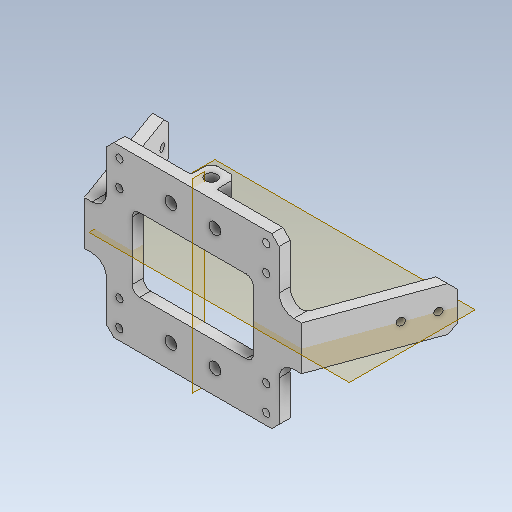
# Autodesk Inventor part: body_shell_2
Saved by Autodesk Inventor 2023 (Build 270158000, 158)
## iProperties
Created: 2021-03-01
Part Number: body_shell_2
Material: Generic
Document SubType Name: Modeling
Designer: Shuang Peng
Density: 1 g/cm^3
Appearance: Default
Author: Shuang Peng
Autodesk Inventor part; units mm, degrees
ref_plane "YZ Plane" through (0, 0, 0) normal (1, 0, 0) x (0, 1, 0)
ref_plane "XZ Plane" through (0, 0, 0) normal (0, 1, 0) x (-1, 0, 0)
ref_plane "XY Plane" through (0, 0, 0) normal (0, 0, 1) x (1, 0, 0)
sketch "Sketch1" plane through (0, 0, 0) normal (0, 0, 1) x (1, 0, 0)
  line L0 (-3.5, 39.5) -> (3.5, 39.5) projected
  line L1 (-3.5, 26.5) -> (-3.5, 39.5) projected
  line L2 (3.5, 26.5) -> (-3.5, 26.5) projected
  line L3 (3.5, 39.5) -> (3.5, 26.5) projected
  circle A0 centre (0, 36.5) radius 1.6 projected
  circle A1 centre (0, 29.5) radius 1.6 projected
  line L4 (-3.5, -6.5) -> (3.5, -6.5) projected
  line L5 (3.5, -6.5) -> (3.5, 6.5) projected
  line L6 (3.5, 6.5) -> (-3.5, 6.5) projected
  line L7 (-3.5, 6.5) -> (-3.5, -6.5) projected
  circle A2 centre (0, -3.5) radius 1.6 projected
  circle A3 centre (0, 3.5) radius 1.6 projected
  line L8 (-36.5, 39.5) -> (-43.5, 39.5) projected
  line L9 (-43.5, 39.5) -> (-43.5, 26.5) projected
  line L10 (-43.5, 26.5) -> (-36.5, 26.5) projected
  line L11 (-36.5, 26.5) -> (-36.5, 39.5) projected
  circle A4 centre (-40, 36.5) radius 1.6 projected
  circle A5 centre (-40, 29.5) radius 1.6 projected
  line L12 (-36.5, -6.5) -> (-43.5, -6.5) projected
  line L13 (-36.5, 6.5) -> (-36.5, -6.5) projected
  line L14 (-43.5, 6.5) -> (-36.5, 6.5) projected
  line L15 (-43.5, -6.5) -> (-43.5, 6.5) projected
  circle A6 centre (-40, -3.5) radius 1.6 projected
  circle A7 centre (-40, 3.5) radius 1.6 projected
  line L16 (3.5, 39.5) -> (-43.5, 39.5)
  line L17 (-43.5, 39.5) -> (-43.5, -6.5)
  line L18 (-43.5, -6.5) -> (3.5, -6.5)
  line L19 (3.5, -6.5) -> (3.5, 39.5)
  line L20 (-3.5, 26.5) -> (-36.5, 26.5)
  line L21 (-36.5, 26.5) -> (-36.5, 6.5)
  line L22 (-36.5, 6.5) -> (-3.5, 6.5)
  line L23 (-3.5, 6.5) -> (-3.5, 26.5)
  point P0 (0, 0)
  constraints: 16 end point, 4 parallel, 2 horizontal, 2 perpendicular
extrude "Extrusion1" add sketch "Sketch1" along normal blind 3 contours L0 L3 L2 L1 | L1 L20 L11 L16 | L2 L19 L6 L23 | L11 L10 L9 L8 | L21 L14 L17 L10 | L6 L5 L4 L7 | L7 L18 L13 L22 | L13 L12 L15 L14 | A0 | A1 | A2 | A3 | A4 | A5 | A6 | A7
sketch "Sketch2" plane through (0, 0, 3) normal (0, 0, 1) x (1, 0, 0)
  circle A0 centre (0, 36.5) radius 1 projected
  circle A1 centre (0, 29.5) radius 1 projected
  circle A2 centre (0, 3.5) radius 1 projected
  circle A3 centre (0, -3.5) radius 1 projected
  circle A4 centre (-40, -3.5) radius 1 projected
  circle A5 centre (-40, 3.5) radius 1 projected
  circle A6 centre (-40, 29.5) radius 1 projected
  circle A7 centre (-40, 36.5) radius 1 projected
  point P0 (0, 0)
hole "Hole1" at (0, 36.5, 3) at (0, 29.5, 3) at (0, 3.5, 3) at (0, -3.5, 3) at (-40, -3.5, 3) at (-40, 3.5, 3) at (-40, 29.5, 3) at (-40, 36.5, 3) direction (0, 0, -1) diameter 2 depth 20
ref_plane "Work Plane1" through (-20, -6.5, 0) normal (1, 0, 0) x (0, 0, -1)
sketch "Sketch3" plane through (0, 0, 0) normal (0, 0, -1) x (-1, 0, 0)
  circle A0 centre (40, 29.5) radius 1 projected
  circle A1 centre (40, -3.5) radius 1 projected
  circle A2 centre (0, 3.5) radius 1 projected
  circle A3 centre (0, 36.5) radius 1 projected
  circle A4 centre (0, 29.5) radius 1 projected
  circle A5 centre (0, -3.5) radius 1 projected
  circle A6 centre (40, 3.5) radius 1 projected
  circle A7 centre (40, 36.5) radius 1 projected
  line L0 (-3.5, 39.5) -> (43.5, 39.5) projected
  line L1 (-3.5, -6.5) -> (-3.5, 39.5) projected
  line L2 (43.5, -6.5) -> (-3.5, -6.5) projected
  line L3 (43.5, 39.5) -> (43.5, -6.5) projected
  line L4 (36.5, 26.5) -> (3.5, 26.5) projected
  line L5 (36.5, 6.5) -> (36.5, 26.5) projected
  line L6 (3.5, 6.5) -> (36.5, 6.5) projected
  line L7 (3.5, 26.5) -> (3.5, 6.5) projected
  line L8 (0.5, 22.5) -> (0.5, 10.5)
  line L9 (0.5, 10.5) -> (-7.5, 10.5)
  line L10 (-7.5, 10.5) -> (-7.5, 22.5)
  line L11 (-7.5, 22.5) -> (0.5, 22.5)
  line L12 (-3.5, -6.5) -> (-3.5, 39.5) projected
  line L13 (0.5, 22.5) -> (-7.5, 10.5) construction
  line L14 (0.5, 10.5) -> (-7.5, 22.5) construction
  point P0 (0, 0)
  point P1 (-3.5, 16.5)
  point P2 (-3.5, 10.5)
  point P3 (-3.5, 22.5)
  dimension "d9" = 12
  dimension "d10" = 8
  constraints: 12 end point, 3 midpoint, 2 parallel, 2 perpendicular
  measures "d9" distance of L8.start L8.end
  measures "d10" distance of L8.end L9.end
extrude "Extrusion2" add sketch "Sketch3" against normal up to surface (3 mm away) contours L1 L9 L10 L11
sketch "Sketch4" plane through (3.5, 10.5, 0) normal (0, -1, 0) x (1, 0, 0)
  line L0 (4, 3) -> (0, 3) projected
  line L1 (0, 0) -> (0, 3) projected
  line L2 (4, 0) -> (0, 0) projected
  line L3 (4, 0) -> (4, 3) projected
  line L4 (4, 0) -> (14.2606, -28.1908)
  line L5 (4, 3) -> (6.1006, 3)
  line L6 (6.1006, 3) -> (17.4531, -28.1908)
  line L7 (17.4531, -28.1908) -> (14.2606, -28.1908)
  point P0 (-3.5, 0)
  dimension "d13" = 30
  dimension "d14" = 110
  dimension "d15" = 3
  constraints: 8 end point, 2 parallel, 1 horizontal
  measures "d13" distance of L2.start L4.end
  measures "d14" angle of L2 L4
  measures "d15" distance between parallel lines of L4 L6
extrude "Extrusion3" add sketch "Sketch4" against normal up to surface (12 mm away) contours L5 L6 L7 L4 L3
ref_plane "Work Plane2" through (17.7606, 16.5, -28.1908) normal (0, 1, 0) x (1, 0, 0)
sketch "Sketch5" plane through (17.7606, 16.5, -28.1908) normal (0, 1, 0) x (1, 0, 0)
  line L0 (-58.7606, -28.1908) -> (-56.7606, -28.1908) projected
  line L1 (-58.7606, -28.1908) -> (-56.7606, -28.1908) projected
  line L2 (-18.7606, -28.1908) -> (-16.7606, -28.1908) projected
  line L3 (-18.7606, -28.1908) -> (-16.7606, -28.1908) projected
  line L4 (-18.7606, -28.1908) -> (-16.7606, -28.1908) projected
  line L5 (-18.7606, -28.1908) -> (-16.7606, -28.1908) projected
  line L6 (-58.7606, -28.1908) -> (-56.7606, -28.1908) projected
  line L7 (-58.7606, -28.1908) -> (-56.7606, -28.1908) projected
  line L8 (-14.2606, -28.1908) -> (-61.2606, -28.1908) projected
  line L9 (-61.2606, -28.1908) -> (-14.2606, -28.1908) projected
  line L10 (-54.2606, -28.1908) -> (-21.2606, -28.1908) projected
  line L11 (-21.2606, -28.1908) -> (-54.2606, -28.1908) projected
  line L12 (-10.2606, -28.1908) -> (0, 0) projected
  line L13 (-10.2606, -28.1908) -> (0, 0) projected
  line L14 (-10.2606, -28.1908) -> (-5.1303, -14.0954)
  line L15 (-21.2606, -28.1908) -> (-21.2606, -31.1908) projected
  line L16 (-5.1303, -14.0954) -> (-21.2606, -28.1908)
  line L17 (-14.2606, -28.1908) -> (-10.2606, -28.1908) projected
  line L18 (-10.2606, -28.1908) -> (-14.2606, -28.1908) projected
  point P0 (-17.7606, -28.1908)
  dimension "d19" = 15
  constraints: 4 end point, 1 midpoint
  measures "d19" distance of L14.start L14.end
extrude "Extrusion4" add sketch "Sketch5" along normal mid plane 2
mirror "Mirror1" about plane through (-20, -6.5, 0) normal (1, 0, 0) of "Extrusion2", "Extrusion3", "Extrusion4"
sketch "Sketch6" plane through (0, 0, 0) normal (0, 0, -1) x (-1, 0, 0)
  line L0 (36.5, 17.5) -> (47.5, 17.5) projected
  line L1 (47.5, 22.5) -> (47.5, 17.5) projected
  line L2 (43.5, 22.5) -> (47.5, 22.5) projected
  line L3 (43.5, 39.5) -> (43.5, 22.5) projected
  line L4 (-3.5, 39.5) -> (43.5, 39.5) projected
  line L5 (-3.5, 22.5) -> (-3.5, 39.5) projected
  line L6 (-3.5, 22.5) -> (-7.5, 22.5) projected
  line L7 (-7.5, 22.5) -> (-7.5, 17.5) projected
  line L8 (-7.5, 17.5) -> (3.5, 17.5) projected
  line L9 (3.5, 26.5) -> (3.5, 17.5) projected
  line L10 (36.5, 26.5) -> (3.5, 26.5) projected
  line L11 (36.5, 17.5) -> (36.5, 26.5) projected
  circle A0 centre (40, 29.5) radius 1 projected
  circle A1 centre (0, 36.5) radius 1 projected
  circle A2 centre (0, 29.5) radius 1 projected
  circle A3 centre (40, 36.5) radius 1 projected
  line L12 (47.5, 15.5) -> (36.5, 15.5) projected
  line L13 (36.5, 6.5) -> (36.5, 15.5) projected
  line L14 (3.5, 6.5) -> (36.5, 6.5) projected
  line L15 (3.5, 15.5) -> (3.5, 6.5) projected
  line L16 (3.5, 15.5) -> (-7.5, 15.5) projected
  line L17 (-7.5, 15.5) -> (-7.5, 10.5) projected
  line L18 (-7.5, 10.5) -> (-3.5, 10.5) projected
  line L19 (-3.5, -6.5) -> (-3.5, 10.5) projected
  line L20 (43.5, -6.5) -> (-3.5, -6.5) projected
  line L21 (43.5, 10.5) -> (43.5, -6.5) projected
  line L22 (47.5, 10.5) -> (43.5, 10.5) projected
  line L23 (47.5, 15.5) -> (47.5, 10.5) projected
  circle A4 centre (40, -3.5) radius 1 projected
  circle A5 centre (0, 3.5) radius 1 projected
  circle A6 centre (0, -3.5) radius 1 projected
  circle A7 centre (40, 3.5) radius 1 projected
  circle A8 centre (40, 36.5) radius 1 projected
  line L24 (40, 36.5) -> (40, 29.5)
  circle A9 centre (0, 36.5) radius 1 projected
  circle A10 centre (0, 29.5) radius 1 projected
  line L25 (0, 36.5) -> (0, 29.5)
  line L26 (40, 33) -> (0, 33)
  line L27 (20, 33) -> (14, 33)
  line L28 (20, 33) -> (26, 33)
  circle A11 centre (26, 33) radius 1.6
  circle A12 centre (14, 33) radius 1.6
  point P0 (0, 0)
  dimension "d23" = 6
  dimension "d24" = 6
  dimension "d25" = 3.2
  dimension "d26" = 3.2
  constraints: 10 end point, 3 midpoint, 2 centre point, 2 coincident, 2 vertical, 1 collinear, 1 point on line
  measures "d23" distance of L27.start L27.end
  measures "d24" distance of L27.start L28.end
  measures "d25" diameter of A11
  measures "d26" diameter of A12
extrude "Extrusion5" cut sketch "Sketch6" against normal blind 6 contours A11 L26 | L26 A11 | A12 L26 | L26 A12
mirror "Mirror2" about plane through (17.7606, 16.5, -28.1908) normal (0, 1, 0) of "Extrusion5"
sketch "Sketch7" plane through (-43.5, 39.5, 0) normal (0, 1, 0) x (1, 0, 0)
  line L0 (47, 0) -> (0, 0) projected
  line L1 (0, 0) -> (0, -3) projected
  line L2 (47, -3) -> (0, -3) projected
  line L3 (47, 0) -> (47, -3) projected
  line L4 (47, 0) -> (0, 0) projected
  line L5 (23.5, 0) -> (23.5, 2)
  line L6 (20, 5.5) -> (20, -1.5)
  line L7 (20, -1.5) -> (27, -1.5)
  line L8 (27, -1.5) -> (27, 5.5)
  line L9 (27, 5.5) -> (20, 5.5)
  line L10 (20, 5.5) -> (27, -1.5) construction
  line L11 (20, -1.5) -> (27, 5.5) construction
  line L12 (7, -3) -> (40, -3) projected
  circle A0 centre (23.5, 2) radius 1.6
  point P0 (43.5, 0)
  point P1 (27, 0)
  point P2 (20, 0)
  dimension "d29" = 2
  dimension "d30" = 7
  dimension "d31" = 7
  dimension "d32" = 3.2
  constraints: 14 end point, 3 midpoint, 2 parallel, 2 perpendicular, 1 centre point, 1 coincident, 1 vertical
  measures "d29" distance of L5.start L5.end
  measures "d30" distance of L6.start L6.end
  measures "d31" distance of L7.end L6.end
  measures "d32" diameter of A0
extrude "Extrusion6" add sketch "Sketch7" against normal blind 6 contours L0 L6 L9 L8
mirror "Mirror3" about plane through (17.7606, 16.5, -28.1908) normal (0, 1, 0) of "Extrusion6"
chamfer "Chamfer1" distance 1.5 angle 45 4 edges at (-23.5, 36.5, -5.5) (-16.5, 36.5, -5.5) (-23.5, -3.5, -5.5) (-16.5, -3.5, -5.5)
fillet "Fillet3" radius 2 2 edges at (-20, 33.5, 0) (-20, -0.5, 0)
fillet "Fillet4" radius 0.5 4 edges at (-23.5, 35.5, 0) (-16.5, 35.5, 0) (-16.5, -2.5, 0) (-23.5, -2.5, 0)
fillet "Fillet5" radius 2 4 edges at (-36.5, 6.5, 1.5) (-3.5, 6.5, 1.5) (-3.5, 26.5, 1.5) (-36.5, 26.5, 1.5)
fillet "Fillet6" radius 2 4 edges at (-47.5, 20, 0) (-47.5, 13, 0) (7.5, 20, 0) (7.5, 13, 0)
fillet "Fillet7" radius 4 4 edges at (-43.5, 22.5, 1.5) (-43.5, 10.5, 1.5) (3.5, 10.5, 1.5) (3.5, 22.5, 1.5)
fillet "Fillet8" radius 1 12 edges at (-47.2467, 17.5, -0.3617) (-41.2998, 17.5, 0) (-50.3046, 17.5, -7.7057) (-47.2467, 15.5, -0.3617) (-41.2998, 15.5, 0) (-50.3046, 15.5, -7.7057) (7.2467, 15.5, -0.3617) (10.3046, 15.5, -7.7057) (1.2998, 15.5, 0) (7.2467, 17.5, -0.3617) (10.3046, 17.5, -7.7057) (1.2998, 17.5, 0)
chamfer "Chamfer2" distance 2 angle 45 4 edges at (-59.3569, 22.5, -28.1908) (-59.3569, 10.5, -28.1908) (19.3569, 22.5, -28.1908) (19.3569, 10.5, -28.1908)
sketch "Sketch8" plane through (-49.6006, 10.5, 3) normal (-0.9396926, 0, 0.3420201) x (0.3420201, 0, 0.9396926)
  circle A0 centre (-29.1006, 6) radius 1.55 projected
  circle A1 centre (-21.1006, 6) radius 1.55 projected
  circle A2 centre (-29.1006, 6) radius 1
  circle A3 centre (-21.1006, 6) radius 1
  point P0 (14.1453, -10.5)
  dimension "d47" = 2
  dimension "d48" = 2
  constraints: 2 centre point, 2 coincident
  measures "d47" diameter of A2
  measures "d48" diameter of A3
extrude "Extrusion7" cut sketch "Sketch8" against normal blind 6 contours A2 | A3
mirror "Mirror4" about plane through (-20, -6.5, 0) normal (1, 0, 0) of "Extrusion7"
chamfer "Chamfer3" distance 2 angle 45 4 edges at (-43.5, -6.5, 1.5) (-43.5, 39.5, 1.5) (3.5, 39.5, 1.5) (3.5, -6.5, 1.5)
body "Solid1"
